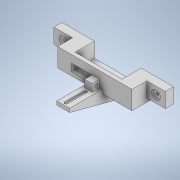
# Autodesk Inventor part: Bottom Bracket + camera bottom thingy
Saved by Autodesk Inventor 2020 (Build 240168000, 168)
## iProperties
Created: 2019-11-12
Part Number: Bottom Bracket + camera bottom thingy
Material: Generic
Document SubType Name: Modeling
Designer: bzs3334
Density: 1 g/cm^3
Appearance: Default
Author: bzs3334
Autodesk Inventor part; units mm, degrees
ref_plane "YZ Plane" through (0, 0, 0) normal (1, 0, 0) x (0, 1, 0)
ref_plane "XZ Plane" through (0, 0, 0) normal (0, 1, 0) x (-1, 0, 0)
ref_plane "XY Plane" through (0, 0, 0) normal (0, 0, 1) x (1, 0, 0)
sketch "Sketch1" plane through (0, 0, 0) normal (0, 1, 0) x (-1, 0, 0)
  line L0 (50, -15.5) -> (-50, -15.5)
  line L1 (-50, -15.5) -> (-50, 15.5)
  line L2 (-50, 15.5) -> (50, 15.5)
  line L3 (50, 15.5) -> (50, -15.5)
  line L4 (31.5, -15.5) -> (-31.5, -15.5)
  line L5 (-31.5, -15.5) -> (-31.5, 10.5)
  line L6 (-31.5, 10.5) -> (31.5, 10.5)
  line L7 (31.5, 10.5) -> (31.5, -15.5)
  line L8 (50, -15.5) -> (75, -15.5)
  line L9 (75, -15.5) -> (75, -4.5)
  line L10 (75, -4.5) -> (50, -4.5)
  line L11 (50, -4.5) -> (50, -15.5)
  line L12 (0, 0) -> (0, -15.5)
  line L13 (-50, -15.5) -> (-75, -15.5)
  line L14 (-75, -15.5) -> (-75, -4.5)
  line L15 (-75, -4.5) -> (-50, -4.5)
  point P0 (-50, -4.5)
  point P1 (-31.5, -15.5)
  dimension "d0" = 100
  dimension "d1" = 50
  dimension "d2" = 31
  dimension "d3" = 15.5
  dimension "d4" = 26
  dimension "d5" = 63
  dimension "d6" = 31.5
  dimension "d7" = 11
  dimension "d8" = 25
  constraints: 32 end point, 6 parallel, 3 horizontal, 3 perpendicular, 3 symmetric about line, 1 midpoint, 1 point on line
  measures "d0" distance of L0.start L0.end
  measures "d1" distance from line of L3 L12.start
  measures "d2" distance of L2.end L0.start
  measures "d3" distance from line of L2 L12.start
  measures "d4" distance of L6.end L4.start
  measures "d5" distance of L5.end L6.end
  measures "d6" distance from line of L5 L12.start
  measures "d7" distance of L8.end L9.end
  measures "d8" distance of L9.end L10.end
extrude "Extrusion1" add sketch "Sketch1" along normal blind 20 contours L0 L7 L6 L5 L1 L2 L3 | L3 L10 L9 L8 | L13 L14 L15 L1
sketch "Sketch2" plane through (-75, 0, -4.5) normal (0, 0, 1) x (1, 0, 0)
  line L0 (0, 0) -> (25, 0) projected
  line L1 (25, 0) -> (25, 20) projected
  line L2 (0, 20) -> (25, 20) projected
  line L3 (0, 0) -> (0, 20) projected
  circle A0 centre (12.5, 10) radius 1.75
  circle A1 centre (12.5, 10) radius 5.75
  point P0 (75, 0)
  dimension "d11" = 3.5
  dimension "d12" = 11.5
  constraints: 2 centre point, 1 coincident
  measures "d11" diameter of A0
  measures "d12" diameter of A1
extrude "Extrusion2" cut sketch "Sketch2" against normal through all contours A0
extrude "Extrusion3" cut sketch "Sketch2" against normal blind 2 contours A1
mirror "Mirror1" about plane through (0, 0, 0) normal (1, 0, 0) of "Extrusion3", "Extrusion2"
sketch "Sketch4" plane through (0, 0, 0) normal (0, -1, 0) x (1, 0, 0)
  line L0 (-31.5, -15.5) -> (-75, -15.5) projected
  line L1 (-31.5, 10.5) -> (-31.5, -15.5) projected
  line L2 (31.5, 10.5) -> (-31.5, 10.5) projected
  line L3 (31.5, -15.5) -> (31.5, 10.5) projected
  line L4 (75, -15.5) -> (31.5, -15.5) projected
  line L5 (75, -4.5) -> (75, -15.5) projected
  line L6 (50, -4.5) -> (75, -4.5) projected
  line L7 (50, 15.5) -> (50, -4.5) projected
  line L8 (-50, 15.5) -> (50, 15.5) projected
  line L9 (-50, -4.5) -> (-50, 15.5) projected
  line L10 (-75, -4.5) -> (-50, -4.5) projected
  line L11 (-75, -15.5) -> (-75, -4.5) projected
  line L12 (75, -15.5) -> (31.5, -15.5) projected
  line L13 (50, -15.5) -> (-50, -15.5)
  line L14 (-50, -15.5) -> (-50, 59.5)
  line L15 (-50, 59.5) -> (50, 59.5)
  line L16 (50, 59.5) -> (50, -15.5)
  point P0 (0, 0)
  dimension "d22" = 100
  dimension "d23" = 75
  constraints: 8 end point, 2 parallel, 1 horizontal, 1 perpendicular, 1 point on line
  measures "d22" distance of L14.end L15.end
  measures "d23" distance of L13.end L14.end
extrude "Extrusion5" add sketch "Sketch4" along normal blind 5 contours L0 L14 L9 L8 L7 L16 L4 L3 L2 L1 | L1 L2 L3 L13 | L14 L15 L16 L8
sketch "Sketch5" plane through (31.5, 20, 10.5) normal (0, 0, -1) x (-1, 0, 0)
  line L0 (63, -20) -> (0, -20) projected
  line L1 (63, -20) -> (35, -20)
  line L2 (35, -20) -> (35, -10)
  line L3 (35, -10) -> (63, -10)
  line L4 (63, -10) -> (63, -20)
  point P0 (31.5, -20)
  dimension "d26" = 28
  dimension "d27" = 10
  constraints: 8 end point, 2 parallel, 1 horizontal, 1 perpendicular
  measures "d26" distance of L2.end L3.end
  measures "d27" distance of L1.end L2.end
extrude "Extrusion6" cut sketch "Sketch5" against normal blind 57
sketch "Sketch7" plane through (0, 0, 0) normal (0, 1, 0) x (1, 0, 0)
  line L0 (-3.5, -10.5) -> (-3.5, -15.5) projected
  line L1 (-50, -15.5) -> (-31.5, -15.5) projected
  line L2 (-50, -59.5) -> (-50, -15.5) projected
  line L3 (50, -59.5) -> (-50, -59.5) projected
  line L4 (50, -15.5) -> (50, -59.5) projected
  line L5 (-3.5, -15.5) -> (50, -15.5) projected
  line L6 (-3.5, -10.5) -> (-3.5, -15.5) projected
  line L7 (31.5, -10.5) -> (-3.5, -10.5) projected
  line L8 (31.5, 15.5) -> (31.5, -10.5) projected
  line L9 (-31.5, 15.5) -> (31.5, 15.5) projected
  line L10 (-31.5, 15.5) -> (-31.5, -15.5) projected
  line L11 (-3.5, -15.5) -> (50, -15.5) projected
  line L12 (50, -59.5) -> (-50, -59.5) projected
  line L13 (-3.5, -15.5) -> (-50, -15.5)
  line L14 (-50, -15.5) -> (-50, -59.5)
  line L15 (-50, -59.5) -> (-3.5, -59.5)
  line L16 (-3.5, -59.5) -> (-3.5, -15.5)
  line L17 (-50, -15.5) -> (50, -15.5) projected
  line L18 (-7.0641, -59.5) -> (-50, -59.5)
  line L19 (-50, -59.5) -> (-50, -15.5)
  line L20 (-50, -15.5) -> (-7.0641, -15.5)
  line L21 (-7.0641, -15.5) -> (-7.0641, -59.5)
  point P0 (0, 0)
  point P1 (-7.0641, -59.5)
  point P2 (-7.0641, -15.5)
  constraints: 16 end point, 4 parallel, 2 horizontal, 2 perpendicular, 1 point on line
extrude "Extrusion8" cut sketch "Sketch7" against normal blind 24.25 contours L21 L3 L2 L1 L13
mirror "Mirror2" about plane through (0, 0, 0) normal (1, 0, 0) of "Extrusion8"
sketch "Sketch11" plane through (0, 0, 0) normal (0, 1, 0) x (1, 0, 0)
  line L0 (7.0641, -59.5) -> (7.0641, -15.5) projected
  line L1 (-3.5, -15.5) -> (7.0641, -15.5) projected
  line L2 (-3.5, -10.5) -> (-3.5, -15.5) projected
  line L3 (31.5, -10.5) -> (-3.5, -10.5) projected
  line L4 (31.5, 15.5) -> (31.5, -10.5) projected
  line L5 (-31.5, 15.5) -> (31.5, 15.5) projected
  line L6 (-31.5, 15.5) -> (-31.5, -15.5) projected
  line L7 (-31.5, -15.5) -> (-7.0641, -15.5) projected
  line L8 (-7.0641, -15.5) -> (-7.0641, -59.5) projected
  line L9 (7.0641, -59.5) -> (-7.0641, -59.5) projected
  line L10 (-3.5, -15.5) -> (3.5, -15.5)
  line L11 (3.5, -15.5) -> (3.5, -20.5)
  line L12 (3.5, -20.5) -> (-3.5, -20.5)
  line L13 (-3.5, -20.5) -> (-3.5, -15.5)
  line L14 (7.0641, -15.5) -> (7.0641, -59.5) projected
  line L15 (7.0641, -20.5) -> (3.5, -20.5)
  point P0 (0, 0)
  point P1 (0, -59.5)
  dimension "d39" = 7
  dimension "d40" = 5
  constraints: 10 end point, 2 parallel, 2 perpendicular, 1 horizontal, 1 midpoint, 1 point on line
  measures "d39" distance of L1.start L10.end
  measures "d40" distance of L10.end L11.end
extrude "Extrusion9" add sketch "Sketch11" along normal blind 10 contours L12 L13 L1 L11
sketch "Sketch16" plane through (-3.5, 0, 20.5) normal (0, 0, 1) x (1, 0, 0)
  line L0 (7, 0) -> (0, 0) projected
  line L1 (7, 0) -> (7, 10) projected
  line L2 (0, 10) -> (7, 10) projected
  line L3 (0, 0) -> (0, 10) projected
  point P0 (3.5, 0)
extrude "Extrusion13" add sketch "Sketch16" along normal blind 5
sketch "Sketch17" plane through (-3.5, 0, 10.5) normal (-1, 0, 0) x (0, 0, 1)
  line L0 (0, 10) -> (5, 10) projected
  line L1 (0, 0) -> (0, 10) projected
  line L2 (15, 0) -> (0, 0) projected
  line L3 (15, 10) -> (15, 0) projected
  line L4 (5, 10) -> (15, 10) projected
  line L5 (5, -5) -> (5, 20) projected
  line L6 (-15, 20) -> (5, 20) projected
  line L7 (-15, 0) -> (-15, 20) projected
  line L8 (-26, 0) -> (-15, 0) projected
  line L9 (-26, 0) -> (-26, -5) projected
  line L10 (5, -5) -> (-26, -5) projected
  circle A0 centre (10, 5) radius 2.1
  point P0 (-10.5, 0)
  dimension "d53" = 5
  dimension "d54" = 4.2
  dimension "d55" = 5
  constraints: 1 centre point
  measures "d53" distance from line of L2 A0.centre
  measures "d54" diameter of A0
  measures "d55" distance from line of L5 A0.centre
sketch "Sketch18" plane through (-7.0641, 0, 15.5) normal (-1, 0, 0) x (0, 0, 1)
  line L0 (44, -5) -> (0, -5) projected
  line L1 (44, 0) -> (44, -5) projected
  line L2 (0, 0) -> (44, 0) projected
  line L3 (0, 0) -> (0, -5) projected
  line L4 (44, -5) -> (0, -5) projected
  line L5 (44, -5) -> (-17.6428, -5)
  line L6 (-31, -5) -> (0, -5) projected
  line L7 (-31, 0) -> (-31, -5) projected
  line L8 (-31, -5) -> (-31, -25)
  line L9 (-31, -25) -> (44, -5)
  point P0 (-15.5, 0)
  point P1 (44, -5)
  point P2 (0, -5)
  dimension "d59" = 20
  dimension "d60" = 75
  constraints: 6 end point, 2 point on line, 1 vertical
  measures "d59" distance of L6.start L8.end
  measures "d60" distance from line of L8 L5.start
extrude "Extrusion15" add sketch "Sketch18" against normal up to surface (14.1282 mm away) contours L9 L8 L6 L5 L0
sketch "Sketch21" plane through (0, 0, 0) normal (0, 1, 0) x (1, 0, 0)
  line L0 (3.5, -15.5) -> (3.5, -25.5) projected
  line L1 (3.5, -25.5) -> (-3.5, -25.5) projected
  line L2 (-3.5, -25.5) -> (-3.5, -10.5) projected
  line L3 (31.5, -10.5) -> (-3.5, -10.5) projected
  line L4 (31.5, 15.5) -> (31.5, -10.5) projected
  line L5 (-31.5, 15.5) -> (31.5, 15.5) projected
  line L6 (-31.5, 15.5) -> (-31.5, -15.5) projected
  line L7 (-31.5, -15.5) -> (-7.0641, -15.5) projected
  line L8 (-7.0641, -15.5) -> (-7.0641, -59.5) projected
  line L9 (7.0641, -59.5) -> (-7.0641, -59.5) projected
  line L10 (7.0641, -59.5) -> (7.0641, -15.5) projected
  line L11 (3.5, -15.5) -> (7.0641, -15.5) projected
  line L12 (7.0641, -59.5) -> (7.0641, -15.5) projected
  line L13 (7.0641, -25.5) -> (3.5, -25.5)
  point P0 (0, 0)
  point P1 (7.0641, -25.5)
  constraints: 2 end point, 1 perpendicular, 1 point on line
extrude "Extrusion16" add sketch "Sketch21" along normal blind 10 contours L11 L10 L13 L0
extrude "Extrusion17" cut sketch "Sketch17" against normal blind 268.25 contours A0
sketch "Sketch22" plane through (7.0641, -5, 15.5) normal (1, 0, 0) x (0, 0, -1)
  circle A0 centre (-5, 10) radius 2.1 projected
  line L0 (0, 15) -> (0, 0) projected
  line L1 (-10, 15) -> (0, 15) projected
  line L2 (-10, 5) -> (-10, 15) projected
  line L3 (-44, 5) -> (-10, 5) projected
  line L4 (-44, 0) -> (-44, 5) projected
  line L5 (-44, 0) -> (31, -20) projected
  line L6 (31, -20) -> (31, 0) projected
  line L7 (0, 0) -> (31, 0) projected
  point P0 (15.5, 5)
extrude "Extrusion18" cut sketch "Sketch22" against normal blind 0.5641
sketch "Sketch25" plane through (6.5, -5, 15.5) normal (1, 0, 0) x (0, 0, -1)
  line L0 (-10, 5) -> (-10, 15) projected
  line L1 (-44, 5) -> (-10, 5) projected
  line L2 (-44, 0) -> (-44, 5) projected
  line L3 (31, -20) -> (-44, 0) projected
  line L4 (31, 0) -> (31, -20) projected
  line L5 (0, 0) -> (31, 0) projected
  line L6 (0, 15) -> (0, 0) projected
  line L7 (-10, 15) -> (0, 15) projected
  circle A0 centre (-5, 10) radius 2.1 projected
  line L8 (-10, 5) -> (5, 5) projected
  line L9 (-10, 5) -> (0, 5)
  point P0 (15.5, 5)
  constraints: 2 end point, 2 point on line
extrude "Extrusion21" add sketch "Sketch25" along normal blind 3.564 contours L8 L6 L5 L4 L3 L2 L1
sketch "Sketch26" plane through (0, 0, 0) normal (0, 1, 0) x (1, 0, 0)
  line L0 (6.5, -25.5) -> (-3.5, -25.5) projected
  line L1 (-3.5, -25.5) -> (-3.5, -10.5) projected
  line L2 (31.5, -10.5) -> (-3.5, -10.5) projected
  line L3 (31.5, 15.5) -> (31.5, -10.5) projected
  line L4 (-31.5, 15.5) -> (31.5, 15.5) projected
  line L5 (-31.5, 15.5) -> (-31.5, -15.5) projected
  line L6 (-31.5, -15.5) -> (-7.0641, -15.5) projected
  line L7 (-7.0641, -15.5) -> (-7.0641, -59.5) projected
  line L8 (10.064, -59.5) -> (-7.0641, -59.5) projected
  line L9 (10.064, -15.5) -> (10.064, -59.5) projected
  line L10 (6.5, -15.5) -> (10.064, -15.5) projected
  line L11 (6.5, -25.5) -> (6.5, -15.5) projected
  line L12 (1.5, -55.5) -> (1.5, -29.5) construction
  line L13 (3.5, -55.5) -> (3.5, -29.5)
  line L14 (-0.5, -29.5) -> (-0.5001, -55.5)
  arc A0 (-0.5001, -55.5) -> (3.5, -55.5) centre (1.5, -55.5) ccw
  arc A1 (3.5, -29.5) -> (-0.5, -29.5) centre (1.5, -29.5) ccw
  point P0 (0, 0)
  point P1 (1.5, -42.5)
  dimension "d77" = 4
  dimension "d78" = 14
  dimension "d79" = 4
  dimension "d80" = 8.564
  constraints: 8 end point, 4 point on circle, 4 tangent, 2 centre point, 1 midpoint, 1 parallel, 1 vertical
  measures "d77" diameter of A1
  measures "d78" distance from line of L10 L12.end
  measures "d79" distance from line of L8 L12.start
  measures "d80" distance between parallel lines of L7 L12
extrude "Extrusion22" cut sketch "Sketch26" against normal blind 2 contours A0 L14 A1 L13
equation "\"d1\" = 0.5 * d0"
equation "\"d3\" = 0.5 * d2"
equation "\"d6\" = 0.5 * d5"
body "Solid1"
